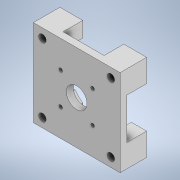
# Autodesk Inventor part: pmtbase
Saved by Autodesk Inventor 2022.2 (Build 262287030, 287C)
## iProperties
Created: 2022-03-11
Part Number: pmtbase
Material: Generic
Document SubType Name: Modeling
Designer: Tapendra
Density: 1 g/cm^3
Appearance: Default
Author: Tapendra
Autodesk Inventor part; units mm, degrees
ref_plane "YZ Plane" through (0, 0, 0) normal (1, 0, 0) x (0, 1, 0)
ref_plane "XZ Plane" through (0, 0, 0) normal (0, 1, 0) x (-1, 0, 0)
ref_plane "XY Plane" through (0, 0, 0) normal (0, 0, 1) x (1, 0, 0)
sketch "Sketch1" plane through (0, 0, 0) normal (0, 0, 1) x (1, 0, 0)
  line L0 (-19, 19) -> (19, 19)
  line L1 (19, 19) -> (19, -19)
  line L2 (19, -19) -> (-19, -19)
  line L3 (-19, -19) -> (-19, 19)
  line L4 (-19, 19) -> (19, -19) construction
  line L5 (19, 19) -> (-19, -19) construction
  circle A0 centre (0, 0) radius 4.5
  dimension "d0" = 38
  dimension "d1" = 38
  dimension "d2" = 9
  constraints: 12 end point, 2 midpoint, 2 parallel, 1 centre point, 1 coincident, 1 horizontal, 1 perpendicular
  measures "d0" distance of L0.end L1.end
  measures "d1" distance of L0.start L0.end
  measures "d2" diameter of A0
extrude "Extrusion1" add sketch "Sketch1" along normal mid plane 11.64
sketch "Sketch4" plane through (0, 0, 5.82) normal (0, 0, 1) x (1, 0, 0)
  line L0 (-11.25, -11.25) -> (11.25, -11.25) construction
  line L1 (11.25, -11.25) -> (11.25, 11.25) construction
  line L2 (11.25, 11.25) -> (-11.25, 11.25) construction
  line L3 (-11.25, 11.25) -> (-11.25, -11.25) construction
  line L4 (-11.25, -11.25) -> (11.25, 11.25) construction
  line L5 (11.25, -11.25) -> (-11.25, 11.25) construction
  point P0 (0, 0)
  point P1 (-7, -7)
  point P2 (0, 0)
  point P3 (0, 0)
  point P4 (-7, 7)
  point P5 (7, -7)
  point P6 (7, 7)
  dimension "d17" = 22.5
  dimension "d18" = 22.5
  dimension "d47" = 7
  dimension "d48" = 7
  dimension "d51" = 14
  dimension "d54" = 14
  constraints: 12 end point, 4 midpoint, 2 horizontal, 2 parallel, 1 perpendicular, 1 vertical, 3 other
  measures "d17" distance of L1.end L2.end
  measures "d18" distance of L2.end L0.start
  measures "d47" horizontal distance of point (-7, -7) point (0, 0)
  measures "d48" horizontal distance of point (-7, -7) point (0, 0)
  measures "d51" distance of point (-7, -7) point (-7, 7)
  measures "d54" distance of point (-7, -7) point (7, -7)
sketch "Sketch5" plane through (0, 0, -5.82) normal (0, 0, -1) x (-1, 0, 0)
  circle A0 centre (0, 0) radius 4.5 projected
  circle A1 centre (0, 0) radius 15.24
  dimension "d19" = 30.48
  constraints: 1 centre point, 1 coincident
  measures "d19" diameter of A1
extrude "Extrusion2" cut sketch "Sketch5" against normal blind 8.64 contours A0 | A1
sketch "Sketch6" plane through (-19, 19, 5.82) normal (0, 1, 0) x (1, 0, 0)
  line L0 (0, 11.64) -> (38, 11.64) projected
  line L1 (3.76, 3) -> (34.24, 3) projected
  line L2 (10, 11.64) -> (28, 11.64)
  line L3 (28, 11.64) -> (28, 3)
  line L4 (28, 3) -> (10, 3)
  line L5 (10, 3) -> (10, 11.64)
  line L6 (0, 11.64) -> (0, 0) projected
  line L7 (38, 11.64) -> (38, 0) projected
  point P0 (19, 5.82)
  point P1 (10, 3)
  dimension "d22" = 10
  dimension "d23" = 10
  constraints: 8 end point, 2 parallel, 2 point on line, 1 horizontal, 1 perpendicular
  measures "d22" distance between parallel lines of L6 L5
  measures "d23" distance between parallel lines of L3 L7
extrude "Extrusion3" cut sketch "Sketch6" against normal through all
sketch "Sketch7" plane through (19, -19, 5.82) normal (1, 0, 0) x (0, 0, -1)
  line L0 (11.64, 31.2987) -> (11.64, 6.7013) projected
  line L1 (3, 31.2987) -> (3, 6.7013) projected
  line L2 (11.64, 28) -> (3, 28)
  line L3 (3, 28) -> (3, 10)
  line L4 (3, 10) -> (11.64, 10)
  line L5 (11.64, 10) -> (11.64, 28)
  line L6 (11.64, 38) -> (0, 38) projected
  line L7 (11.64, 0) -> (0, 0) projected
  point P0 (5.82, 19)
  point P1 (11.64, 10)
  point P2 (3, 28)
  dimension "d26" = 10
  dimension "d27" = 10
  constraints: 8 end point, 2 parallel, 2 point on line, 1 horizontal, 1 perpendicular
  measures "d26" distance between parallel lines of L2 L6
  measures "d27" distance between parallel lines of L7 L4
extrude "Extrusion4" cut sketch "Sketch7" against normal through all
sketch "Sketch8" plane through (0, 0, -5.82) normal (0, 0, -1) x (-1, 0, 0)
  line L0 (-12.2987, -9) -> (-19, -9) projected
  line L1 (-19, -9) -> (-19, -19) projected
  line L2 (-19, -19) -> (-9, -19) projected
  line L3 (-9, -19) -> (-9, -12.2987) projected
  arc A0 (-12.2987, -9) -> (-9, -12.2987) centre (0, 0) ccw projected
  point P0 (-15, -15)
  point P1 (-15, 15)
  point P2 (15, -15)
  point P3 (15, 15)
  dimension "d30" = 15
  dimension "d31" = 15
  dimension "d34" = 30
  dimension "d37" = 30
  constraints: 1 horizontal, 1 vertical, 3 other
  measures "d30" horizontal distance of point (-15, -15) point (0, 0)
  measures "d31" horizontal distance of point (-15, -15) point (0, 0)
  measures "d34" distance of point (-15, -15) point (-15, 15)
  measures "d37" distance of point (-15, -15) point (15, -15)
hole "Hole1" at (15, -15, -5.82) at (15, 15, -5.82) at (-15, 15, -5.82) at (-15, -15, -5.82) direction (0, 0, 1) diameter 3.242 depth 4 thread size "M4x0.7" class "6H" standard "ANSI Metric M Profile"
hole "Hole2" at (-7, -7, 5.82) at (-7, 7, 5.82) at (7, -7, 5.82) at (7, 7, 5.82) direction (0, 0, -1) diameter 1.567 end through all thread size "M2x0.4" class "6H" standard "ANSI Metric M Profile"
sketch "Sketch9" plane through (0, 0, 5.82) normal (0, 0, 1) x (1, 0, 0)
  circle A0 centre (15, -15) radius 1.621 projected
  circle A1 centre (-15, -15) radius 1.621 projected
  circle A2 centre (-15, 15) radius 1.621 projected
  circle A3 centre (15, 15) radius 1.621 projected
  point P0 (0, 0)
  constraints: 4 coincident
hole "Hole3" at (15, -15, 5.82) at (-15, -15, 5.82) at (-15, 15, 5.82) at (15, 15, 5.82) direction (0, 0, -1) diameter 3.242 end through all thread size "M4x0.7" class "6H" standard "ANSI Metric M Profile"
equation "\"d1\" = d0"
equation "\"d18\" = d17"
body "Solid1"
